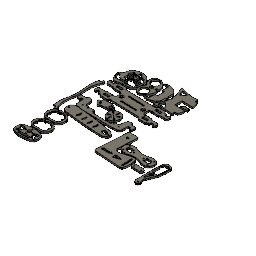
cat (Autodesk Fusion 360 design; units mm, degrees)
Autodesk Fusion 360 part; units mm, degrees
note: some values were not read from the file. Set by a fixed rule: which sketch regions a step uses.
(part 1 of 8)
sketch "Sketch1" plane through (0, 0, 0) normal (0, 1, 0) x (1, 0, 0)
  spline S0 degree 3 poles (30.1007, -167.9411) (18.5284, -167.6813) (11.3297, -174.7657) (11.4241, -183.0193) knots 0 0 0 0 1 1 1 1
  spline S1 degree 2 poles (11.4241, -183.0193) (11.5507, -194.1027) (22.4385, -196.859) knots 0 0 0 1 1 1
  line L0 (22.4385, -196.859) -> (39.1149, -197.0671)
  spline S2 degree 2 poles (39.1149, -197.0671) (49.0605, -194.4346) (48.8809, -182.6793) knots 0 0 0 1 1 1
  spline S3 degree 3 poles (48.8809, -182.6793) (48.7831, -176.2778) (41.5132, -168.2292) (30.1007, -167.9411) knots 0 0 0 0 1 1 1 1
  spline S4 degree 2 poles (16.3262, -186.15) (16.3682, -187.7873) (16.3594, -188.6061) knots 0 0 0 1 1 1
  spline S5 degree 3 poles (16.3594, -188.6061) (16.3555, -188.96) (16.5341, -189.4138) (17.0331, -189.4233) knots 0 0 0 0 1 1 1 1
  spline S6 degree 2 poles (17.0331, -189.4233) (17.5465, -189.433) (18.5735, -189.4411) knots 0 0 0 1 1 1
  spline S7 degree 2 poles (18.5735, -189.4411) (18.5349, -191.4596) (18.5681, -192.6548) knots 0 0 0 1 1 1
  spline S8 degree 3 poles (18.5681, -192.6548) (18.5726, -192.8153) (18.7396, -193.0355) (18.9408, -193.0336) knots 0 0 0 0 1 1 1 1
  spline S9 degree 3 poles (18.9408, -193.0336) (20.2717, -193.0206) (33.282, -192.9942) (40.4733, -192.9561) knots 0 0 0 0 1 1 1 1
  spline S10 degree 3 poles (40.4733, -192.9561) (40.6565, -192.9551) (40.8487, -192.7855) (40.8532, -192.6394) knots 0 0 0 0 1 1 1 1
  spline S11 degree 3 poles (40.8532, -192.6394) (40.8827, -191.6807) (40.867, -191.3134) (40.8652, -190.4928) knots 0 0 0 0 1 1 1 1
  spline S12 degree 3 poles (40.8652, -190.4928) (40.8648, -190.322) (41.0647, -190.1082) (41.2786, -190.1006) knots 0 0 0 0 1 1 1 1
  spline S13 degree 2 poles (41.2786, -190.1006) (41.9764, -190.0758) (43.3093, -190.0656) knots 0 0 0 1 1 1
  line L1 (43.3093, -190.0656) -> (43.2511, -186.7175)
  spline S14 degree 2 poles (43.2511, -186.7175) (41.3833, -185.9275) (41.4303, -183.8853) knots 0 0 0 1 1 1
  spline S15 degree 2 poles (41.4303, -183.8853) (41.4654, -182.3626) (43.665, -181.4955) knots 0 0 0 1 1 1
  line L2 (43.665, -181.4955) -> (43.6777, -178.3696)
  line L3 (43.6777, -178.3696) -> (41.9176, -178.351)
  spline S16 degree 3 poles (41.9176, -178.351) (41.6673, -178.3482) (41.388, -178.1253) (41.3891, -177.9256) knots 0 0 0 0 1 1 1 1
  line L4 (41.3891, -177.9256) -> (41.4058, -175.2138)
  spline S17 degree 3 poles (41.4058, -175.2138) (41.4074, -174.9545) (41.0839, -174.6323) (40.7588, -174.6317) knots 0 0 0 0 1 1 1 1
  line L5 (40.7588, -174.6317) -> (37.4248, -174.625)
  spline S18 degree 2 poles (37.4248, -174.625) (37.4304, -174.643) (37.4477, -173.8298) knots 0 0 0 1 1 1
  spline S19 degree 3 poles (37.4477, -173.8298) (37.4575, -173.3685) (37.471, -172.6397) (37.4893, -171.4884) knots 0 0 0 0 1 1 1 1
  spline S20 degree 3 poles (37.4893, -171.4884) (37.4915, -171.3464) (37.2058, -171.2102) (37.0279, -171.2118) knots 0 0 0 0 1 1 1 1
  spline S21 degree 3 poles (37.0279, -171.2118) (34.0609, -171.2378) (29.7217, -171.2387) (28.7942, -171.2468) knots 0 0 0 0 1 1 1 1
  spline S22 degree 3 poles (28.7942, -171.2468) (28.592, -171.2487) (28.1312, -171.3775) (28.1295, -171.5388) knots 0 0 0 0 1 1 1 1
  spline S23 degree 3 poles (28.1295, -171.5388) (28.1098, -173.3866) (28.1519, -172.4662) (28.1098, -173.3866) knots 0 0 0 0 1 1 1 1
  spline S24 degree 3 poles (28.1098, -173.3866) (28.0952, -173.7064) (27.5382, -174.0379) (27.2259, -174.0384) knots 0 0 0 0 1 1 1 1
  spline S25 degree 3 poles (27.2259, -174.0384) (25.0158, -174.0422) (22.0838, -174.0194) (20.0803, -174.0317) knots 0 0 0 0 1 1 1 1
  spline S26 degree 3 poles (20.0803, -174.0317) (19.6876, -174.0346) (19.3849, -174.3251) (19.3885, -174.6384) knots 0 0 0 0 1 1 1 1
  spline S27 degree 3 poles (19.3885, -174.6384) (19.3931, -175.0333) (19.3962, -176.3013) (19.4093, -176.8891) knots 0 0 0 0 1 1 1 1
  spline S28 degree 3 poles (19.4093, -176.8891) (19.4223, -177.4769) (19.0429, -177.3787) (18.7383, -177.3844) knots 0 0 0 0 1 1 1 1
  spline S29 degree 3 poles (18.7383, -177.3844) (18.0475, -177.3973) (17.5642, -177.4064) (17.2536, -177.4122) knots 0 0 0 0 1 1 1 1
  spline S30 degree 3 poles (17.2536, -177.4122) (16.943, -177.4179) (16.8656, -177.5739) (16.8603, -177.7204) knots 0 0 0 0 1 1 1 1
  spline S31 degree 2 poles (16.8603, -177.7204) (16.8284, -178.6066) (16.8714, -179.9909) knots 0 0 0 1 1 1
  spline S32 degree 3 poles (16.8714, -179.9909) (18.5933, -180.665) (18.7033, -181.7831) (18.7467, -183.0137) knots 0 0 0 0 1 1 1 1
  spline S33 degree 3 poles (18.7467, -183.0137) (18.7915, -184.2826) (18.3153, -185.8023) (16.3262, -186.15) knots 0 0 0 0 1 1 1 1
  spline S34 degree 3 poles (16.5132, -182.6529) (15.9028, -182.6481) (15.6342, -183.0282) (15.649, -183.3882) knots 0 0 0 0 1 1 1 1
  spline S35 degree 3 poles (15.649, -183.3882) (15.6637, -183.749) (15.9951, -184.0326) (16.5484, -184.0283) knots 0 0 0 0 1 1 1 1
  spline S36 degree 3 poles (16.5484, -184.0283) (17.0419, -184.0245) (17.3667, -183.6763) (17.3661, -183.3666) knots 0 0 0 0 1 1 1 1
  spline S37 degree 3 poles (17.3661, -183.3666) (17.3652, -182.9178) (16.9336, -182.6565) (16.5132, -182.6529) knots 0 0 0 0 1 1 1 1
  spline S38 degree 3 poles (43.0664, -183.5551) (42.456, -183.5503) (42.1875, -183.9304) (42.2022, -184.2904) knots 0 0 0 0 1 1 1 1
  spline S39 degree 3 poles (42.2022, -184.2904) (42.217, -184.6513) (42.5483, -184.9349) (43.1016, -184.9305) knots 0 0 0 0 1 1 1 1
  spline S40 degree 3 poles (43.1016, -184.9305) (43.5952, -184.9267) (43.9199, -184.5786) (43.9193, -184.2688) knots 0 0 0 0 1 1 1 1
  spline S41 degree 3 poles (43.9193, -184.2688) (43.9185, -183.8201) (43.4868, -183.5587) (43.0664, -183.5551) knots 0 0 0 0 1 1 1 1
  spline S42 degree 3 poles (23.7842, -171.0421) (22.7975, -171.0345) (22.3635, -171.6745) (22.3872, -172.281) knots 0 0 0 0 1 1 1 1
  spline S43 degree 3 poles (22.3872, -172.281) (22.4111, -172.889) (22.9467, -173.3668) (23.8411, -173.3594) knots 0 0 0 0 1 1 1 1
  spline S44 degree 3 poles (23.8411, -173.3594) (24.6388, -173.3528) (25.1637, -172.7664) (25.1628, -172.2446) knots 0 0 0 0 1 1 1 1
  spline S45 degree 3 poles (25.1628, -172.2446) (25.1615, -171.4885) (24.4637, -171.0481) (23.7842, -171.0421) knots 0 0 0 0 1 1 1 1
  spline S46 degree 3 poles (197.2264, -186.8151) (204.2093, -186.9093) (204.3289, -186.987) (213.7082, -187.3044) knots 0 0 0 0 1 1 1 1
  spline S47 degree 3 poles (213.7082, -187.3044) (214.9527, -187.2349) (217.7236, -188.5503) (217.578, -192.0838) knots 0 0 0 0 1 1 1 1
  spline S48 degree 3 poles (217.578, -192.0838) (217.428, -195.7284) (214.5453, -196.5174) (213.4322, -196.3773) knots 0 0 0 0 1 1 1 1
  spline S49 degree 3 poles (213.4322, -196.3773) (204.6722, -196.078) (204.6859, -195.9838) (197.5085, -195.7356) knots 0 0 0 0 1 1 1 1
  spline S50 degree 3 poles (197.5085, -195.7356) (196.2722, -195.7521) (193.3363, -194.4697) (193.4517, -191.1659) knots 0 0 0 0 1 1 1 1
  spline S51 degree 3 poles (193.4517, -191.1659) (193.5843, -187.3752) (195.8081, -186.9513) (197.2264, -186.8151) knots 0 0 0 0 1 1 1 1
  spline S52 degree 3 poles (197.9729, -187.867) (199.884, -187.9236) (201.1067, -189.5978) (201.0786, -191.1557) knots 0 0 0 0 1 1 1 1
  spline S53 degree 3 poles (201.0786, -191.1557) (201.0504, -192.8262) (199.5544, -194.4019) (197.7982, -194.3846) knots 0 0 0 0 1 1 1 1
  spline S54 degree 3 poles (197.7982, -194.3846) (196.0791, -194.3681) (194.5964, -192.8234) (194.5755, -191.0496) knots 0 0 0 0 1 1 1 1
  spline S55 degree 3 poles (194.5755, -191.0496) (194.5553, -189.4029) (195.9362, -187.8065) (197.9729, -187.867) knots 0 0 0 0 1 1 1 1
  spline S56 degree 3 poles (197.8992, -188.8932) (199.2233, -188.9345) (200.0706, -190.1307) (200.051, -191.2446) knots 0 0 0 0 1 1 1 1
  spline S57 degree 3 poles (200.051, -191.2446) (200.0267, -192.4391) (198.9949, -193.5657) (197.7781, -193.5533) knots 0 0 0 0 1 1 1 1
  spline S58 degree 3 poles (197.7781, -193.5533) (196.5871, -193.5409) (195.5596, -192.4371) (195.5452, -191.1688) knots 0 0 0 0 1 1 1 1
  spline S59 degree 3 poles (195.5452, -191.1688) (195.529, -189.9915) (196.4879, -188.85) (197.8992, -188.8932) knots 0 0 0 0 1 1 1 1
  spline S60 degree 3 poles (212.9873, -188.7216) (214.8985, -188.7782) (216.1212, -190.4524) (216.0931, -192.0102) knots 0 0 0 0 1 1 1 1
  spline S61 degree 3 poles (216.0931, -192.0102) (216.0648, -193.6808) (214.5689, -195.2565) (212.8127, -195.2392) knots 0 0 0 0 1 1 1 1
  spline S62 degree 3 poles (212.8127, -195.2392) (211.0936, -195.2227) (209.6108, -193.678) (209.59, -191.9042) knots 0 0 0 0 1 1 1 1
  spline S63 degree 3 poles (209.59, -191.9042) (209.5698, -190.2575) (210.9506, -188.6611) (212.9873, -188.7216) knots 0 0 0 0 1 1 1 1
  spline S64 degree 3 poles (212.9137, -189.7478) (214.2378, -189.7891) (215.0851, -190.9853) (215.0655, -192.0992) knots 0 0 0 0 1 1 1 1
  spline S65 degree 3 poles (215.0655, -192.0992) (215.0412, -193.2937) (214.0094, -194.4203) (212.7926, -194.4079) knots 0 0 0 0 1 1 1 1
  spline S66 degree 3 poles (212.7926, -194.4079) (211.6015, -194.3955) (210.5741, -193.2917) (210.5596, -192.0234) knots 0 0 0 0 1 1 1 1
  spline S67 degree 3 poles (210.5596, -192.0234) (210.5435, -190.8461) (211.5024, -189.7046) (212.9137, -189.7478) knots 0 0 0 0 1 1 1 1
  spline S68 degree 3 poles (197.9022, -190.3368) (198.3782, -190.3493) (198.6826, -190.771) (198.6756, -191.1619) knots 0 0 0 0 1 1 1 1
  spline S69 degree 3 poles (198.6756, -191.1619) (198.6674, -191.581) (198.296, -191.9763) (197.8586, -191.972) knots 0 0 0 0 1 1 1 1
  spline S70 degree 3 poles (197.8586, -191.972) (197.4305, -191.969) (197.0612, -191.5805) (197.056, -191.1353) knots 0 0 0 0 1 1 1 1
  spline S71 degree 3 poles (197.056, -191.1353) (197.0479, -190.7223) (197.3951, -190.3217) (197.9022, -190.3368) knots 0 0 0 0 1 1 1 1
  spline S72 degree 3 poles (212.9168, -191.2402) (213.3928, -191.2526) (213.6972, -191.6744) (213.6902, -192.0653) knots 0 0 0 0 1 1 1 1
  spline S73 degree 3 poles (213.6902, -192.0653) (213.682, -192.4843) (213.3106, -192.8796) (212.8732, -192.8753) knots 0 0 0 0 1 1 1 1
  spline S74 degree 3 poles (212.8732, -192.8753) (212.4451, -192.8723) (212.0758, -192.4838) (212.0706, -192.0386) knots 0 0 0 0 1 1 1 1
  spline S75 degree 3 poles (212.0706, -192.0386) (212.0625, -191.6256) (212.4097, -191.2251) (212.9168, -191.2402) knots 0 0 0 0 1 1 1 1
  line L6 (146.865, -211.1125) -> (145.6182, -211.0016)
  spline S76 degree 3 poles (145.6182, -211.0016) (143.5328, -215.233) (142.4397, -219.9965) (142.4613, -224.7587) knots 0 0 0 0 1 1 1 1
  spline S77 degree 3 poles (142.4613, -224.7587) (142.4822, -229.3508) (143.5381, -233.9343) (145.519, -238.0307) knots 0 0 0 0 1 1 1 1
  line L7 (145.519, -238.0307) -> (146.5081, -237.9343)
  line L8 (146.5081, -237.9343) -> (147.1109, -234.9727)
  line L9 (147.1109, -234.9727) -> (150.1451, -235.1898)
  line L10 (150.1451, -235.1898) -> (150.4167, -238.3519)
  spline S78 degree 3 poles (150.4167, -238.3519) (151.2044, -238.3226) (151.9926, -238.3081) (152.7808, -238.3082) knots 0 0 0 0 1 1 1 1
  spline S79 degree 3 poles (152.7808, -238.3082) (155.0336, -238.3085) (157.3099, -238.4326) (159.4772, -239.077) knots 0 0 0 0 1 1 1 1
  spline S80 degree 3 poles (159.4772, -239.077) (162.8464, -240.0787) (165.767, -242.276) (168.9964, -243.6958) knots 0 0 0 0 1 1 1 1
  spline S81 degree 3 poles (168.9964, -243.6958) (172.6327, -245.2945) (176.6166, -245.8823) (180.56, -245.9048) knots 0 0 0 0 1 1 1 1
  spline S82 degree 3 poles (180.56, -245.9048) (184.3344, -245.9265) (188.147, -245.4327) (191.6764, -244.0305) knots 0 0 0 0 1 1 1 1
  spline S83 degree 3 poles (191.6764, -244.0305) (195.8908, -242.3562) (199.6632, -239.411) (204.0862, -238.5023) knots 0 0 0 0 1 1 1 1
  spline S84 degree 3 poles (204.0862, -238.5023) (205.3946, -238.2335) (206.7377, -238.1508) (208.0672, -238.2572) knots 0 0 0 0 1 1 1 1
  line L11 (208.0672, -238.2572) -> (210.3957, -238.4357)
  line L12 (210.3957, -238.4357) -> (210.8097, -235.2303)
  line L13 (210.8097, -235.2303) -> (213.5445, -235.2773)
  line L14 (213.5445, -235.2773) -> (214.0524, -237.8947)
  line L15 (214.0524, -237.8947) -> (215.7016, -237.8617)
  spline S85 degree 3 poles (215.7016, -237.8617) (216.1906, -236.8171) (216.6159, -235.7396) (216.9738, -234.6382) knots 0 0 0 0 1 1 1 1
  spline S86 degree 3 poles (216.9738, -234.6382) (218.027, -231.3975) (218.4906, -227.9675) (218.5697, -224.5451) knots 0 0 0 0 1 1 1 1
  spline S87 degree 3 poles (218.5697, -224.5451) (218.6361, -221.6728) (218.4324, -218.7783) (217.7433, -215.9974) knots 0 0 0 0 1 1 1 1
  spline S88 degree 3 poles (217.7433, -215.9974) (217.3137, -214.2641) (216.6969, -212.5818) (215.9083, -210.993) knots 0 0 0 0 1 1 1 1
  line L16 (215.9083, -210.993) -> (214.1259, -211.0241)
  line L17 (214.1259, -211.0241) -> (213.9265, -214.1277)
  line L18 (213.9265, -214.1277) -> (210.6322, -213.958)
  spline S89 degree 3 poles (210.6322, -213.958) (210.5729, -213.3726) (210.5658, -212.7815) (210.611, -212.1948) knots 0 0 0 0 1 1 1 1
  spline S90 degree 3 poles (210.611, -212.1948) (210.6283, -211.9695) (210.6533, -211.743) (210.6307, -211.5182) knots 0 0 0 0 1 1 1 1
  spline S91 degree 3 poles (210.6307, -211.5182) (210.608, -211.2935) (210.5323, -211.0664) (210.3768, -210.9098) knots 0 0 0 0 1 1 1 1
  spline S92 degree 3 poles (210.3768, -210.9098) (210.2363, -210.7684) (210.0354, -210.6956) (209.8416, -210.7158) knots 0 0 0 0 1 1 1 1
  spline S93 degree 3 poles (209.8416, -210.7158) (209.6478, -210.736) (209.4646, -210.8489) (209.3535, -211.0165) knots 0 0 0 0 1 1 1 1
  spline S94 degree 3 poles (209.3535, -211.0165) (206.6023, -213.213) (202.9, -214.0441) (199.5315, -213.2216) knots 0 0 0 0 1 1 1 1
  spline S95 degree 3 poles (199.5315, -213.2216) (197.267, -212.6687) (195.2184, -211.4328) (193.0787, -210.4795) knots 0 0 0 0 1 1 1 1
  spline S96 degree 3 poles (193.0787, -210.4795) (189.1673, -208.737) (184.8924, -207.9308) (180.6427, -208.0084) knots 0 0 0 0 1 1 1 1
  spline S97 degree 3 poles (180.6427, -208.0084) (176.3537, -208.0868) (172.1019, -209.0544) (168.0772, -210.6096) knots 0 0 0 0 1 1 1 1
  spline S98 degree 3 poles (168.0772, -210.6096) (164.8763, -211.8464) (161.7028, -213.4776) (158.2919, -213.5448) knots 0 0 0 0 1 1 1 1
  spline S99 degree 3 poles (158.2919, -213.5448) (156.5255, -213.5795) (154.6945, -213.1518) (153.3097, -212.0024) knots 0 0 0 0 1 1 1 1
  spline S100 degree 3 poles (153.3097, -212.0024) (153.0083, -211.7523) (152.7298, -211.4699) (152.4066, -211.2518) knots 0 0 0 0 1 1 1 1
  spline S101 degree 3 poles (152.4066, -211.2518) (152.0833, -211.0337) (151.7007, -210.8809) (151.3189, -210.9292) knots 0 0 0 0 1 1 1 1
  spline S102 degree 3 poles (151.3189, -210.9292) (151.021, -210.9669) (150.7394, -211.1305) (150.5511, -211.3753) knots 0 0 0 0 1 1 1 1
  spline S103 degree 3 poles (150.5511, -211.3753) (150.3629, -211.6201) (150.2701, -211.9432) (150.2982, -212.2562) knots 0 0 0 0 1 1 1 1
  line L19 (150.2982, -212.2562) -> (150.1937, -214.0445)
  line L20 (150.1937, -214.0445) -> (146.9587, -214.0134)
  line L21 (146.9587, -214.0134) -> (146.865, -211.1125)
  line L22 (175.7677, -213.3062) -> (185.4169, -213.3732)
  spline S104 degree 3 poles (185.4169, -213.3732) (185.5698, -213.3654) (185.7249, -213.4272) (185.8333, -213.5405) knots 0 0 0 0 1 1 1 1
  spline S105 degree 3 poles (185.8333, -213.5405) (185.9415, -213.6536) (186.0014, -213.8157) (185.9941, -213.9756) knots 0 0 0 0 1 1 1 1
  line L23 (185.9941, -213.9756) -> (185.9941, -235.4239)
  spline S106 degree 3 poles (185.9941, -235.4239) (185.9786, -235.596) (185.9102, -235.7625) (185.8013, -235.8925) knots 0 0 0 0 1 1 1 1
  spline S107 degree 3 poles (185.8013, -235.8925) (185.6858, -236.0305) (185.5252, -236.1263) (185.353, -236.1602) knots 0 0 0 0 1 1 1 1
  line L24 (185.353, -236.1602) -> (175.8327, -235.9594)
  spline S108 degree 3 poles (175.8327, -235.9594) (175.6725, -235.8987) (175.5277, -235.7938) (175.4169, -235.6581) knots 0 0 0 0 1 1 1 1
  spline S109 degree 3 poles (175.4169, -235.6581) (175.3008, -235.516) (175.2225, -235.3405) (175.1927, -235.1561) knots 0 0 0 0 1 1 1 1
  line L25 (175.1927, -235.1561) -> (175.1608, -213.9224)
  spline S110 degree 3 poles (175.1608, -213.9224) (175.1845, -213.7836) (175.2461, -213.652) (175.3365, -213.5474) knots 0 0 0 0 1 1 1 1
  spline S111 degree 3 poles (175.3365, -213.5474) (175.448, -213.4183) (175.6033, -213.3315) (175.7677, -213.3062) knots 0 0 0 0 1 1 1 1
  line L26 (163.9244, -228.8555) -> (163.9212, -233.8159)
  spline S112 degree 3 poles (163.9212, -233.8159) (163.875, -234.1512) (163.9842, -234.5062) (164.2085, -234.7502) knots 0 0 0 0 1 1 1 1
  spline S113 degree 3 poles (164.2085, -234.7502) (164.3318, -234.8843) (164.4876, -234.9853) (164.6572, -235.041) knots 0 0 0 0 1 1 1 1
  spline S114 degree 3 poles (164.6572, -235.041) (164.8268, -235.0967) (165.0097, -235.107) (165.184, -235.0706) knots 0 0 0 0 1 1 1 1
  line L27 (165.184, -235.0706) -> (171.8437, -235.1161)
  spline S115 degree 3 poles (171.8437, -235.1161) (172.1006, -235.0921) (172.345, -234.9471) (172.4969, -234.7287) knots 0 0 0 0 1 1 1 1
  spline S116 degree 3 poles (172.4969, -234.7287) (172.6109, -234.5648) (172.6729, -234.3619) (172.6711, -234.1591) knots 0 0 0 0 1 1 1 1
  line L28 (172.6711, -234.1591) -> (172.6914, -228.797)
  spline S117 degree 3 poles (172.6914, -228.797) (172.692, -228.6495) (172.6925, -228.5015) (172.6735, -228.3554) knots 0 0 0 0 1 1 1 1
  spline S118 degree 3 poles (172.6735, -228.3554) (172.6542, -228.2093) (172.6138, -228.064) (172.5361, -227.941) knots 0 0 0 0 1 1 1 1
  spline S119 degree 3 poles (172.5361, -227.941) (172.465, -227.8286) (172.3636, -227.7375) (172.2466, -227.6812) knots 0 0 0 0 1 1 1 1
  spline S120 degree 3 poles (172.2466, -227.6812) (172.1296, -227.6249) (171.9975, -227.6037) (171.8698, -227.6206) knots 0 0 0 0 1 1 1 1
  line L29 (171.8698, -227.6206) -> (164.5904, -227.6875)
  spline S121 degree 3 poles (164.5904, -227.6875) (164.3694, -227.7576) (164.1743, -227.9139) (164.0518, -228.1191) knots 0 0 0 0 1 1 1 1
  spline S122 degree 3 poles (164.0518, -228.1191) (163.9225, -228.3357) (163.8758, -228.605) (163.9244, -228.8555) knots 0 0 0 0 1 1 1 1
  line L30 (187.9184, -228.9748) -> (188.0011, -233.9299)
  spline S123 degree 3 poles (188.0011, -233.9299) (188.0279, -234.2742) (188.1865, -234.6053) (188.4341, -234.8334) knots 0 0 0 0 1 1 1 1
  spline S124 degree 3 poles (188.4341, -234.8334) (188.6573, -235.039) (188.9502, -235.1598) (189.2473, -235.1688) knots 0 0 0 0 1 1 1 1
  line L31 (189.2473, -235.1688) -> (196.0874, -235.1491)
  spline S125 degree 3 poles (196.0874, -235.1491) (196.4065, -235.1391) (196.7165, -234.9587) (196.8928, -234.6798) knots 0 0 0 0 1 1 1 1
  spline S126 degree 3 poles (196.8928, -234.6798) (196.9656, -234.5647) (197.0157, -234.4345) (197.0428, -234.2994) knots 0 0 0 0 1 1 1 1
  spline S127 degree 3 poles (197.0428, -234.2994) (197.0699, -234.1643) (197.073, -234.0254) (197.0735, -233.8873) knots 0 0 0 0 1 1 1 1
  line L32 (197.0735, -233.8873) -> (197.0923, -228.9078)
  spline S128 degree 3 poles (197.0923, -228.9078) (197.0727, -228.5996) (196.9287, -228.3023) (196.7028, -228.1038) knots 0 0 0 0 1 1 1 1
  spline S129 degree 3 poles (196.7028, -228.1038) (196.5063, -227.9312) (196.2504, -227.8342) (195.9939, -227.8354) knots 0 0 0 0 1 1 1 1
  line L33 (195.9939, -227.8354) -> (188.9046, -227.8076)
  spline S130 degree 3 poles (188.9046, -227.8076) (188.7383, -227.801) (188.5704, -227.8396) (188.4227, -227.9201) knots 0 0 0 0 1 1 1 1
  spline S131 degree 3 poles (188.4227, -227.9201) (188.275, -228.0006) (188.1479, -228.122) (188.0579, -228.2688) knots 0 0 0 0 1 1 1 1
  spline S132 degree 3 poles (188.0579, -228.2688) (187.9312, -228.4756) (187.8805, -228.7322) (187.9184, -228.9748) knots 0 0 0 0 1 1 1 1
  line L34 (170.0186, -222.2752) -> (162.7994, -223.1454)
  spline S133 degree 3 poles (162.7994, -223.1454) (162.5278, -223.1766) (162.2457, -223.0903) (162.0327, -222.911) knots 0 0 0 0 1 1 1 1
  spline S134 degree 3 poles (162.0327, -222.911) (161.8968, -222.7967) (161.789, -222.6459) (161.7224, -222.4772) knots 0 0 0 0 1 1 1 1
  spline S135 degree 3 poles (161.7224, -222.4772) (161.6557, -222.3084) (161.6304, -222.122) (161.6494, -221.9404) knots 0 0 0 0 1 1 1 1
  line L35 (161.6494, -221.9404) -> (161.4651, -219.7207)
  spline S136 degree 3 poles (161.4651, -219.7207) (161.4358, -219.4894) (161.4927, -219.2472) (161.6212, -219.0566) knots 0 0 0 0 1 1 1 1
  spline S137 degree 3 poles (161.6212, -219.0566) (161.7857, -218.8127) (162.0671, -218.6601) (162.3522, -218.6604) knots 0 0 0 0 1 1 1 1
  line L36 (162.3522, -218.6604) -> (169.316, -217.6563)
  spline S138 degree 3 poles (169.316, -217.6563) (169.6522, -217.6146) (170.0024, -217.7125) (170.2742, -217.9241) knots 0 0 0 0 1 1 1 1
  spline S139 degree 3 poles (170.2742, -217.9241) (170.5631, -218.1489) (170.7593, -218.5001) (170.8051, -218.874) knots 0 0 0 0 1 1 1 1
  line L37 (170.8051, -218.874) -> (170.8732, -220.9866)
  spline S140 degree 3 poles (170.8732, -220.9866) (170.8785, -221.2891) (170.7825, -221.5925) (170.6057, -221.8317) knots 0 0 0 0 1 1 1 1
  spline S141 degree 3 poles (170.6057, -221.8317) (170.4559, -222.0343) (170.2494, -222.1903) (170.0186, -222.2752) knots 0 0 0 0 1 1 1 1
  line L38 (198.197, -223.3422) -> (191.3245, -221.9128)
  spline S142 degree 3 poles (191.3245, -221.9128) (191.0607, -221.8499) (190.821, -221.6821) (190.6647, -221.4508) knots 0 0 0 0 1 1 1 1
  spline S143 degree 3 poles (190.6647, -221.4508) (190.4638, -221.1537) (190.4074, -220.7548) (190.5174, -220.4095) knots 0 0 0 0 1 1 1 1
  line L39 (190.5174, -220.4095) -> (190.8221, -218.2444)
  spline S144 degree 3 poles (190.8221, -218.2444) (190.8379, -218.0208) (190.9439, -217.8057) (191.1088, -217.6628) knots 0 0 0 0 1 1 1 1
  spline S145 degree 3 poles (191.1088, -217.6628) (191.2127, -217.5728) (191.3388, -217.511) (191.4714, -217.4853) knots 0 0 0 0 1 1 1 1
  spline S146 degree 3 poles (191.4714, -217.4853) (191.604, -217.4595) (191.7429, -217.4698) (191.8707, -217.515) knots 0 0 0 0 1 1 1 1
  line L40 (191.8707, -217.515) -> (198.5352, -218.7375)
  spline S147 degree 3 poles (198.5352, -218.7375) (198.8622, -218.8129) (199.1617, -219.0127) (199.3654, -219.2912) knots 0 0 0 0 1 1 1 1
  spline S148 degree 3 poles (199.3654, -219.2912) (199.5853, -219.5919) (199.6906, -219.982) (199.6536, -220.3589) knots 0 0 0 0 1 1 1 1
  line L41 (199.6536, -220.3589) -> (199.2644, -222.3859)
  spline S149 degree 3 poles (199.2644, -222.3859) (199.2116, -222.6695) (199.0558, -222.9307) (198.8356, -223.1046) knots 0 0 0 0 1 1 1 1
  spline S150 degree 3 poles (198.8356, -223.1046) (198.6524, -223.2494) (198.4262, -223.3335) (198.197, -223.3422) knots 0 0 0 0 1 1 1 1
  spline S151 degree 3 poles (177.8923, -243.2372) (178.0147, -243.3291) (178.1552, -243.3939) (178.3018, -243.4299) knots 0 0 0 0 1 1 1 1
  spline S152 degree 3 poles (178.3018, -243.4299) (178.4484, -243.4659) (178.6001, -243.4715) (178.7507, -243.474) knots 0 0 0 0 1 1 1 1
  line L42 (178.7507, -243.474) -> (181.8525, -243.5228)
  spline S153 degree 3 poles (181.8525, -243.5228) (182.2174, -243.5104) (182.5745, -243.3344) (182.8164, -243.048) knots 0 0 0 0 1 1 1 1
  spline S154 degree 3 poles (182.8164, -243.048) (183.0715, -242.746) (183.1936, -242.3239) (183.1352, -241.9253) knots 0 0 0 0 1 1 1 1
  spline S155 degree 3 poles (183.1352, -241.9253) (183.0769, -241.5267) (182.8371, -241.1603) (182.5002, -240.9653) knots 0 0 0 0 1 1 1 1
  spline S156 degree 3 poles (182.5002, -240.9653) (182.255, -240.8234) (181.963, -240.7724) (181.687, -240.8233) knots 0 0 0 0 1 1 1 1
  line L43 (181.687, -240.8233) -> (178.6725, -240.775)
  spline S157 degree 3 poles (178.6725, -240.775) (178.5266, -240.7728) (178.3792, -240.7755) (178.2379, -240.8133) knots 0 0 0 0 1 1 1 1
  spline S158 degree 3 poles (178.2379, -240.8133) (178.0966, -240.8512) (177.9639, -240.9211) (177.8472, -241.0127) knots 0 0 0 0 1 1 1 1
  spline S159 degree 3 poles (177.8472, -241.0127) (177.5162, -241.2721) (177.3152, -241.7042) (177.324, -242.1371) knots 0 0 0 0 1 1 1 1
  spline S160 degree 3 poles (177.324, -242.1371) (177.3325, -242.5701) (177.5511, -242.9928) (177.8923, -243.2372) knots 0 0 0 0 1 1 1 1
  spline S161 degree 3 poles (180.3317, -237.7466) (180.0656, -237.7578) (179.7785, -238.083) (179.7896, -238.3619) knots 0 0 0 0 1 1 1 1
  spline S162 degree 3 poles (179.7896, -238.3619) (179.8002, -238.6185) (180.0866, -238.883) (180.3317, -238.8825) knots 0 0 0 0 1 1 1 1
  spline S163 degree 3 poles (180.3317, -238.8825) (180.5981, -238.8821) (180.919, -238.5937) (180.919, -238.3146) knots 0 0 0 0 1 1 1 1
  spline S164 degree 3 poles (180.919, -238.3146) (180.919, -238.0354) (180.5979, -237.7354) (180.3317, -237.7466) knots 0 0 0 0 1 1 1 1
  spline S165 degree 3 poles (180.5804, -210.3406) (180.3142, -210.3518) (180.0272, -210.677) (180.0383, -210.9559) knots 0 0 0 0 1 1 1 1
  spline S166 degree 3 poles (180.0383, -210.9559) (180.0489, -211.2125) (180.3353, -211.477) (180.5804, -211.4766) knots 0 0 0 0 1 1 1 1
  spline S167 degree 3 poles (180.5804, -211.4766) (180.8468, -211.4761) (181.1677, -211.1877) (181.1677, -210.9086) knots 0 0 0 0 1 1 1 1
  spline S168 degree 3 poles (181.1677, -210.9086) (181.1677, -210.6295) (180.8466, -210.3294) (180.5804, -210.3406) knots 0 0 0 0 1 1 1 1
  spline S169 degree 3 poles (87.8377, -110.5872) (84.4918, -110.7696) (81.236, -112.3681) (79.0016, -114.9427) knots 0 0 0 0 1 1 1 1
  spline S170 degree 3 poles (79.0016, -114.9427) (76.7673, -117.5174) (75.5862, -121.0383) (75.8169, -124.4851) knots 0 0 0 0 1 1 1 1
  spline S171 degree 3 poles (75.8169, -124.4851) (76.0391, -127.8061) (77.5645, -131.0121) (79.9651, -133.2378) knots 0 0 0 0 1 1 1 1
  spline S172 degree 3 poles (79.9651, -133.2378) (82.3657, -135.4635) (85.6124, -136.6872) (88.8395, -136.5989) knots 0 0 0 0 1 1 1 1
  spline S173 degree 3 poles (88.8395, -136.5989) (92.1214, -136.509) (95.3527, -135.0611) (97.6441, -132.6368) knots 0 0 0 0 1 1 1 1
  spline S174 degree 3 poles (97.6441, -132.6368) (99.9355, -130.2124) (101.2572, -126.8374) (101.2246, -123.4522) knots 0 0 0 0 1 1 1 1
  spline S175 degree 3 poles (101.2246, -123.4522) (101.1908, -119.9384) (99.6936, -116.468) (97.1968, -114.0765) knots 0 0 0 0 1 1 1 1
  spline S176 degree 3 poles (97.1968, -114.0765) (94.7, -111.6849) (91.2408, -110.4016) (87.8377, -110.5872) knots 0 0 0 0 1 1 1 1
  line L44 (84.5138, -120.8698) -> (80.3813, -118.6573)
  spline S177 degree 3 poles (80.3813, -118.6573) (80.0801, -118.4223) (79.8836, -118.05) (79.8558, -117.6616) knots 0 0 0 0 1 1 1 1
  spline S178 degree 3 poles (79.8558, -117.6616) (79.828, -117.2732) (79.9692, -116.8752) (80.2336, -116.5971) knots 0 0 0 0 1 1 1 1
  spline S179 degree 3 poles (80.2336, -116.5971) (80.4902, -116.3272) (80.8585, -116.1741) (81.225, -116.185) knots 0 0 0 0 1 1 1 1
  spline S180 degree 3 poles (81.225, -116.185) (81.5914, -116.196) (81.9505, -116.3707) (82.1916, -116.6555) knots 0 0 0 0 1 1 1 1
  line L45 (82.1916, -116.6555) -> (84.9102, -120.3218)
  spline S181 degree 3 poles (84.9102, -120.3218) (84.9596, -120.3668) (84.9955, -120.4273) (85.012, -120.4931) knots 0 0 0 0 1 1 1 1
  spline S182 degree 3 poles (85.012, -120.4931) (85.0284, -120.5589) (85.0254, -120.6297) (85.0032, -120.6937) knots 0 0 0 0 1 1 1 1
  spline S183 degree 3 poles (85.0032, -120.6937) (84.97, -120.79) (84.8929, -120.869) (84.7994, -120.9026) knots 0 0 0 0 1 1 1 1
  spline S184 degree 3 poles (84.7994, -120.9026) (84.7058, -120.9362) (84.5978, -120.9239) (84.5138, -120.8698) knots 0 0 0 0 1 1 1 1
  spline S185 degree 3 poles (95.6513, -128.1996) (95.9444, -128.379) (96.165, -128.6802) (96.2523, -129.0199) knots 0 0 0 0 1 1 1 1
  spline S186 degree 3 poles (96.2523, -129.0199) (96.3396, -129.3597) (96.2926, -129.734) (96.1241, -130.0396) knots 0 0 0 0 1 1 1 1
  spline S187 degree 3 poles (96.1241, -130.0396) (95.9293, -130.393) (95.5731, -130.647) (95.1836, -130.7103) knots 0 0 0 0 1 1 1 1
  spline S188 degree 3 poles (95.1836, -130.7103) (94.7941, -130.7737) (94.3795, -130.6448) (94.0887, -130.3703) knots 0 0 0 0 1 1 1 1
  line L46 (94.0887, -130.3703) -> (91.2541, -126.7052)
  spline S189 degree 3 poles (91.2541, -126.7052) (91.2029, -126.6418) (91.1738, -126.5599) (91.173, -126.4774) knots 0 0 0 0 1 1 1 1
  spline S190 degree 3 poles (91.173, -126.4774) (91.1723, -126.395) (91.2, -126.3125) (91.25, -126.2481) knots 0 0 0 0 1 1 1 1
  spline S191 degree 3 poles (91.25, -126.2481) (91.3094, -126.1718) (91.3999, -126.1222) (91.4945, -126.1141) knots 0 0 0 0 1 1 1 1
  spline S192 degree 3 poles (91.4945, -126.1141) (91.589, -126.1064) (91.6863, -126.1397) (91.757, -126.205) knots 0 0 0 0 1 1 1 1
  line L47 (91.757, -126.205) -> (95.6513, -128.1996)
  spline S193 degree 3 poles (95.9911, -119.2601) (96.2564, -119.0604) (96.6058, -118.9842) (96.9269, -119.0559) knots 0 0 0 0 1 1 1 1
  spline S194 degree 3 poles (96.9269, -119.0559) (97.2479, -119.1276) (97.5354, -119.3461) (97.6969, -119.6411) knots 0 0 0 0 1 1 1 1
  spline S195 degree 3 poles (97.6969, -119.6411) (97.8559, -119.9317) (97.8903, -120.2917) (97.7895, -120.6087) knots 0 0 0 0 1 1 1 1
  spline S196 degree 3 poles (97.7895, -120.6087) (97.6886, -120.9257) (97.454, -121.1947) (97.159, -121.3316) knots 0 0 0 0 1 1 1 1
  line L48 (97.159, -121.3316) -> (92.6906, -122.4058)
  spline S197 degree 3 poles (92.6906, -122.4058) (92.6145, -122.4329) (92.5295, -122.4329) (92.4534, -122.4057) knots 0 0 0 0 1 1 1 1
  spline S198 degree 3 poles (92.4534, -122.4057) (92.3772, -122.3785) (92.3104, -122.3244) (92.2669, -122.2545) knots 0 0 0 0 1 1 1 1
  spline S199 degree 3 poles (92.2669, -122.2545) (92.2231, -122.1844) (92.2031, -122.0989) (92.2109, -122.016) knots 0 0 0 0 1 1 1 1
  spline S200 degree 3 poles (92.2109, -122.016) (92.2187, -121.933) (92.2543, -121.8531) (92.3103, -121.793) knots 0 0 0 0 1 1 1 1
  line L49 (92.3103, -121.793) -> (95.9911, -119.2601)
  spline S201 degree 3 poles (80.0987, -128.1123) (79.8187, -128.2317) (79.4945, -128.2368) (79.211, -128.1264) knots 0 0 0 0 1 1 1 1
  spline S202 degree 3 poles (79.211, -128.1264) (78.9275, -128.0159) (78.6876, -127.791) (78.554, -127.5105) knots 0 0 0 0 1 1 1 1
  spline S203 degree 3 poles (78.554, -127.5105) (78.4007, -127.1885) (78.3916, -126.7971) (78.5297, -126.4678) knots 0 0 0 0 1 1 1 1
  spline S204 degree 3 poles (78.5297, -126.4678) (78.6678, -126.1386) (78.9507, -125.8774) (79.2833, -125.7721) knots 0 0 0 0 1 1 1 1
  line L50 (79.2833, -125.7721) -> (83.8434, -124.8303)
  spline S205 degree 3 poles (83.8434, -124.8303) (83.9215, -124.7935) (84.013, -124.7877) (84.0948, -124.8145) knots 0 0 0 0 1 1 1 1
  spline S206 degree 3 poles (84.0948, -124.8145) (84.1766, -124.8413) (84.2481, -124.9004) (84.2912, -124.977) knots 0 0 0 0 1 1 1 1
  spline S207 degree 3 poles (84.2912, -124.977) (84.3347, -125.0543) (84.3489, -125.1487) (84.3302, -125.2359) knots 0 0 0 0 1 1 1 1
  spline S208 degree 3 poles (84.3302, -125.2359) (84.3114, -125.3233) (84.2599, -125.4025) (84.1888, -125.4536) knots 0 0 0 0 1 1 1 1
  line L51 (84.1888, -125.4536) -> (80.0987, -128.1123)
  line L52 (88.6963, -119.2519) -> (88.675, -114.4028)
  spline S209 degree 3 poles (88.675, -114.4028) (88.6406, -114.0553) (88.7574, -113.6949) (88.9875, -113.4385) knots 0 0 0 0 1 1 1 1
  spline S210 degree 3 poles (88.9875, -113.4385) (89.2176, -113.1822) (89.5571, -113.0343) (89.8957, -113.0428) knots 0 0 0 0 1 1 1 1
  spline S211 degree 3 poles (89.8957, -113.0428) (90.2902, -113.0527) (90.6737, -113.2784) (90.8826, -113.6236) knots 0 0 0 0 1 1 1 1
  spline S212 degree 3 poles (90.8826, -113.6236) (91.0916, -113.9689) (91.1196, -114.4233) (90.9549, -114.7931) knots 0 0 0 0 1 1 1 1
  line L53 (90.9549, -114.7931) -> (89.5024, -119.3859)
  spline S213 degree 3 poles (89.5024, -119.3859) (89.4846, -119.4831) (89.4322, -119.5733) (89.3575, -119.6355) knots 0 0 0 0 1 1 1 1
  spline S214 degree 3 poles (89.3575, -119.6355) (89.2828, -119.6976) (89.1863, -119.7313) (89.0903, -119.7287) knots 0 0 0 0 1 1 1 1
  spline S215 degree 3 poles (89.0903, -119.7287) (88.9762, -119.7254) (88.8643, -119.6705) (88.7902, -119.5809) knots 0 0 0 0 1 1 1 1
  spline S216 degree 3 poles (88.7902, -119.5809) (88.7162, -119.4913) (88.6811, -119.3687) (88.6963, -119.2519) knots 0 0 0 0 1 1 1 1
  spline S217 degree 3 poles (87.8977, -127.9601) (87.9089, -129.4698) (87.9162, -130.9795) (87.9196, -132.4893) knots 0 0 0 0 1 1 1 1
  spline S218 degree 3 poles (87.9196, -132.4893) (87.9274, -132.8282) (87.7934, -133.1682) (87.5586, -133.4055) knots 0 0 0 0 1 1 1 1
  spline S219 degree 3 poles (87.5586, -133.4055) (87.3238, -133.6429) (86.9916, -133.7742) (86.6631, -133.7595) knots 0 0 0 0 1 1 1 1
  spline S220 degree 3 poles (86.6631, -133.7595) (86.292, -133.7429) (85.9332, -133.538) (85.7227, -133.2224) knots 0 0 0 0 1 1 1 1
  spline S221 degree 3 poles (85.7227, -133.2224) (85.5123, -132.9068) (85.4551, -132.488) (85.5728, -132.1247) knots 0 0 0 0 1 1 1 1
  line L54 (85.5728, -132.1247) -> (87.0679, -127.8349)
  spline S222 degree 3 poles (87.0679, -127.8349) (87.0929, -127.7408) (87.1495, -127.6561) (87.2258, -127.5985) knots 0 0 0 0 1 1 1 1
  spline S223 degree 3 poles (87.2258, -127.5985) (87.3021, -127.5409) (87.3975, -127.5109) (87.492, -127.5147) knots 0 0 0 0 1 1 1 1
  spline S224 degree 3 poles (87.492, -127.5147) (87.6014, -127.5191) (87.7083, -127.5694) (87.7832, -127.6517) knots 0 0 0 0 1 1 1 1
  spline S225 degree 3 poles (87.7832, -127.6517) (87.8581, -127.734) (87.9001, -127.8471) (87.8977, -127.9601) knots 0 0 0 0 1 1 1 1
  spline S226 degree 3 poles (88.2976, -123.1479) (88.1746, -123.1402) (88.0492, -123.1865) (87.9591, -123.2731) knots 0 0 0 0 1 1 1 1
  spline S227 degree 3 poles (87.9591, -123.2731) (87.8691, -123.3598) (87.8155, -123.4856) (87.8147, -123.6127) knots 0 0 0 0 1 1 1 1
  spline S228 degree 3 poles (87.8147, -123.6127) (87.8139, -123.724) (87.8532, -123.8352) (87.9234, -123.9198) knots 0 0 0 0 1 1 1 1
  spline S229 degree 3 poles (87.9234, -123.9198) (87.9936, -124.0044) (88.0942, -124.0616) (88.201, -124.0775) knots 0 0 0 0 1 1 1 1
  spline S230 degree 3 poles (88.201, -124.0775) (88.3292, -124.0966) (88.4646, -124.055) (88.5619, -123.967) knots 0 0 0 0 1 1 1 1
  spline S231 degree 3 poles (88.5619, -123.967) (88.6593, -123.879) (88.717, -123.7462) (88.7162, -123.6127) knots 0 0 0 0 1 1 1 1
  spline S232 degree 3 poles (88.7162, -123.6127) (88.7155, -123.4966) (88.6713, -123.3814) (88.5947, -123.2963) knots 0 0 0 0 1 1 1 1
  spline S233 degree 3 poles (88.5947, -123.2963) (88.518, -123.2112) (88.4099, -123.1572) (88.2976, -123.1479) knots 0 0 0 0 1 1 1 1
  line L55 (145.2588, -33.5908) -> (147.4545, -33.5908)
  line L56 (147.4545, -33.5908) -> (147.4545, -34.5936)
  spline S234 degree 3 poles (147.4545, -34.5936) (147.4426, -34.7069) (147.4761, -34.8243) (147.5459, -34.9144) knots 0 0 0 0 1 1 1 1
  spline S235 degree 3 poles (147.5459, -34.9144) (147.6304, -35.0236) (147.7677, -35.0901) (147.9058, -35.0889) knots 0 0 0 0 1 1 1 1
  line L57 (147.9058, -35.0889) -> (150.9762, -35.0807)
  spline S236 degree 3 poles (150.9762, -35.0807) (151.1407, -35.0795) (151.3039, -35.0163) (151.4262, -34.9063) knots 0 0 0 0 1 1 1 1
  spline S237 degree 3 poles (151.4262, -34.9063) (151.56, -34.786) (151.6429, -34.6103) (151.6509, -34.4307) knots 0 0 0 0 1 1 1 1
  line L58 (151.6509, -34.4307) -> (151.6322, -33.5782)
  line L59 (151.6322, -33.5782) -> (153.2632, -33.5415)
  line L60 (153.2632, -33.5415) -> (155.0015, -39.4872)
  line L61 (155.0015, -39.4872) -> (140.4552, -39.4147)
  line L62 (140.4552, -39.4147) -> (145.2585, -33.5893)
  line L63 (145.2585, -33.5893) -> (145.2588, -33.5908)
  spline S238 degree 3 poles (152.9413, -139.0973) (153.0574, -138.5407) (152.8687, -137.9469) (152.4352, -137.5051) knots 0 0 0 0 1 1 1 1
  spline S239 degree 3 poles (152.4352, -137.5051) (152.0733, -137.1363) (151.5471, -136.8757) (150.9771, -136.783) knots 0 0 0 0 1 1 1 1
  line L64 (150.9771, -136.783) -> (134.7351, -136.4507)
  spline S240 degree 3 poles (134.7351, -136.4507) (134.1896, -136.3913) (133.6161, -136.5275) (133.1964, -136.816) knots 0 0 0 0 1 1 1 1
  spline S241 degree 3 poles (133.1964, -136.816) (132.9356, -136.9952) (132.7339, -137.2302) (132.6173, -137.4907) knots 0 0 0 0 1 1 1 1
  spline S242 degree 3 poles (132.6173, -137.4907) (132.5008, -137.7512) (132.4698, -138.0364) (132.5282, -138.3095) knots 0 0 0 0 1 1 1 1
  line L65 (132.5282, -138.3095) -> (128.64, -202.1235)
  spline S243 degree 3 poles (128.64, -202.1235) (128.6631, -202.7447) (128.9206, -203.359) (129.3692, -203.8632) knots 0 0 0 0 1 1 1 1
  spline S244 degree 3 poles (129.3692, -203.8632) (129.8461, -204.3993) (130.5375, -204.808) (131.3132, -205.0122) knots 0 0 0 0 1 1 1 1
  line L66 (131.3132, -205.0122) -> (185.3432, -208.5574)
  spline S245 degree 3 poles (185.3432, -208.5574) (186.5202, -208.7117) (187.7794, -208.3694) (188.6035, -207.6712) knots 0 0 0 0 1 1 1 1
  spline S246 degree 3 poles (188.6035, -207.6712) (189.0837, -207.2644) (189.4179, -206.7457) (189.5555, -206.1939) knots 0 0 0 0 1 1 1 1
  spline S247 degree 3 poles (189.5555, -206.1939) (191.833, -198.9698) (192.2769, -191.3695) (190.8515, -184.0034) knots 0 0 0 0 1 1 1 1
  spline S248 degree 3 poles (190.8515, -184.0034) (190.588, -182.6414) (190.2528, -181.2667) (189.4827, -180.0374) knots 0 0 0 0 1 1 1 1
  spline S249 degree 3 poles (189.4827, -180.0374) (189.0977, -179.4228) (188.6044, -178.8491) (187.9905, -178.372) knots 0 0 0 0 1 1 1 1
  spline S250 degree 3 poles (187.9905, -178.372) (187.3766, -177.8949) (186.6397, -177.516) (185.8292, -177.3069) knots 0 0 0 0 1 1 1 1
  spline S251 degree 3 poles (185.8292, -177.3069) (184.7984, -177.0409) (183.6823, -177.0562) (182.6184, -177.2149) knots 0 0 0 0 1 1 1 1
  spline S252 degree 3 poles (182.6184, -177.2149) (181.5544, -177.3737) (180.5306, -177.6707) (179.5109, -177.9634) knots 0 0 0 0 1 1 1 1
  spline S253 degree 3 poles (179.5109, -177.9634) (174.1099, -179.5135) (168.6705, -180.9739) (163.229, -182.4277) knots 0 0 0 0 1 1 1 1
  spline S254 degree 3 poles (163.229, -182.4277) (161.8093, -182.807) (160.381, -183.1875) (158.9025, -183.3662) knots 0 0 0 0 1 1 1 1
  spline S255 degree 3 poles (158.9025, -183.3662) (157.424, -183.5448) (155.8785, -183.5131) (154.4804, -183.0843) knots 0 0 0 0 1 1 1 1
  spline S256 degree 3 poles (154.4804, -183.0843) (153.3104, -182.7254) (152.266, -182.0854) (151.5642, -181.2461) knots 0 0 0 0 1 1 1 1
  spline S257 degree 3 poles (151.5642, -181.2461) (150.7386, -180.2587) (150.4116, -179.0058) (150.6732, -177.8321) knots 0 0 0 0 1 1 1 1
  line L67 (150.6732, -177.8321) -> (152.9413, -139.0973)
  line L68 (141.8092, -151.153) -> (144.1576, -148.9711)
  spline S258 degree 3 poles (144.1576, -148.9711) (144.3427, -148.737) (144.4014, -148.4397) (144.3157, -148.1706) knots 0 0 0 0 1 1 1 1
  spline S259 degree 3 poles (144.3157, -148.1706) (144.23, -147.9014) (144.0011, -147.6642) (143.6994, -147.532) knots 0 0 0 0 1 1 1 1
  spline S260 degree 3 poles (143.6994, -147.532) (143.3474, -147.3777) (142.9025, -147.3719) (142.5445, -147.5169) knots 0 0 0 0 1 1 1 1
  spline S261 degree 3 poles (142.5445, -147.5169) (142.1866, -147.662) (141.9253, -147.954) (141.8665, -148.2748) knots 0 0 0 0 1 1 1 1
  spline S262 degree 3 poles (141.8665, -148.2748) (141.849, -148.1147) (141.7807, -147.9584) (141.6702, -147.825) knots 0 0 0 0 1 1 1 1
  spline S263 degree 3 poles (141.6702, -147.825) (141.5596, -147.6915) (141.4069, -147.5812) (141.2307, -147.5075) knots 0 0 0 0 1 1 1 1
  spline S264 degree 3 poles (141.2307, -147.5075) (141.0545, -147.4338) (140.8551, -147.3968) (140.6569, -147.4011) knots 0 0 0 0 1 1 1 1
  spline S265 degree 3 poles (140.6569, -147.4011) (140.4587, -147.405) (140.262, -147.4508) (140.0908, -147.532) knots 0 0 0 0 1 1 1 1
  spline S266 degree 3 poles (140.0908, -147.532) (139.8003, -147.6698) (139.589, -147.9125) (139.5261, -148.1805) knots 0 0 0 0 1 1 1 1
  spline S267 degree 3 poles (139.5261, -148.1805) (139.4633, -148.4485) (139.5501, -148.7372) (139.7581, -148.9517) knots 0 0 0 0 1 1 1 1
  line L69 (139.7581, -148.9517) -> (141.8092, -151.153)
  spline S268 degree 3 poles (172.7469, -194.5735) (172.9307, -194.4863) (173.0796, -194.3515) (173.1661, -194.1938) knots 0 0 0 0 1 1 1 1
  spline S269 degree 3 poles (173.1661, -194.1938) (173.2525, -194.036) (173.2763, -193.8561) (173.2329, -193.6872) knots 0 0 0 0 1 1 1 1
  spline S270 degree 3 poles (173.2329, -193.6872) (173.1892, -193.5169) (173.0776, -193.3586) (172.9188, -193.2417) knots 0 0 0 0 1 1 1 1
  spline S271 degree 3 poles (172.9188, -193.2417) (172.7601, -193.1247) (172.5551, -193.0497) (172.3418, -193.0306) knots 0 0 0 0 1 1 1 1
  line L70 (172.3418, -193.0306) -> (161.5277, -190.7984)
  spline S272 degree 3 poles (161.5277, -190.7984) (161.281, -190.7505) (161.018, -190.7587) (160.7765, -190.822) knots 0 0 0 0 1 1 1 1
  spline S273 degree 3 poles (160.7765, -190.822) (160.5351, -190.8853) (160.316, -191.0035) (160.1506, -191.1595) knots 0 0 0 0 1 1 1 1
  spline S274 degree 3 poles (160.1506, -191.1595) (159.9749, -191.3253) (159.8607, -191.5335) (159.8266, -191.7504) knots 0 0 0 0 1 1 1 1
  line L71 (159.8266, -191.7504) -> (159.7456, -197.0928)
  spline S275 degree 3 poles (159.7456, -197.0928) (159.7601, -197.4387) (160.0025, -197.773) (160.3684, -197.9514) knots 0 0 0 0 1 1 1 1
  spline S276 degree 3 poles (160.3684, -197.9514) (160.5665, -198.0481) (160.7973, -198.1003) (161.0286, -198.1008) knots 0 0 0 0 1 1 1 1
  spline S277 degree 3 poles (161.0286, -198.1008) (161.2598, -198.1013) (161.4909, -198.0501) (161.6898, -197.9544) knots 0 0 0 0 1 1 1 1
  line L72 (161.6898, -197.9544) -> (172.7469, -194.5735)
  spline S278 degree 3 poles (134.2076, -194.4583) (135.0439, -194.804) (136.0062, -194.8821) (136.9441, -194.9155) knots 0 0 0 0 1 1 1 1
  spline S279 degree 3 poles (136.9441, -194.9155) (137.582, -194.9382) (138.221, -194.9431) (138.8593, -194.93) knots 0 0 0 0 1 1 1 1
  line L73 (138.8593, -194.93) -> (139.7185, -193.9551)
  line L74 (139.7185, -193.9551) -> (140.5491, -195.0229)
  spline S280 degree 3 poles (140.5491, -195.0229) (142.4682, -195.0355) (144.3878, -195.0123) (146.3056, -194.9532) knots 0 0 0 0 1 1 1 1
  spline S281 degree 3 poles (146.3056, -194.9532) (147.5238, -194.9157) (148.7462, -194.8633) (149.9428, -194.6747) knots 0 0 0 0 1 1 1 1
  spline S282 degree 3 poles (149.9428, -194.6747) (151.1099, -194.4907) (152.2673, -194.168) (153.2083, -193.5791) knots 0 0 0 0 1 1 1 1
  spline S283 degree 3 poles (153.2083, -193.5791) (153.5103, -193.3901) (153.796, -193.1651) (153.9335, -192.8767) knots 0 0 0 0 1 1 1 1
  spline S284 degree 3 poles (153.9335, -192.8767) (154.0023, -192.7324) (154.0314, -192.5743) (154.0023, -192.4215) knots 0 0 0 0 1 1 1 1
  spline S285 degree 3 poles (154.0023, -192.4215) (153.9732, -192.2687) (153.8837, -192.1219) (153.7415, -192.0189) knots 0 0 0 0 1 1 1 1
  spline S286 degree 3 poles (153.7415, -192.0189) (153.5718, -191.8961) (153.3298, -191.8421) (153.1065, -191.8771) knots 0 0 0 0 1 1 1 1
  line L75 (153.1065, -191.8771) -> (151.0844, -191.981)
  line L76 (151.0844, -191.981) -> (151.0361, -190.6811)
  line L77 (151.0361, -190.6811) -> (150.3763, -190.3748)
  spline S287 degree 3 poles (150.3763, -190.3748) (150.2527, -190.3515) (150.1185, -190.3679) (150.0085, -190.4186) knots 0 0 0 0 1 1 1 1
  spline S288 degree 3 poles (150.0085, -190.4186) (149.8625, -190.4864) (149.7634, -190.6163) (149.7537, -190.7524) knots 0 0 0 0 1 1 1 1
  line L78 (149.7537, -190.7524) -> (149.8286, -192.6088)
  line L79 (149.8286, -192.6088) -> (147.6696, -192.6224)
  line L80 (147.6696, -192.6224) -> (147.5808, -191.4243)
  line L81 (147.5808, -191.4243) -> (147.2802, -191.1733)
  spline S289 degree 3 poles (147.2802, -191.1733) (147.2057, -191.111) (147.1332, -191.0469) (147.0521, -190.9901) knots 0 0 0 0 1 1 1 1
  spline S290 degree 3 poles (147.0521, -190.9901) (146.9711, -190.9334) (146.8765, -190.8848) (146.7705, -190.8726) knots 0 0 0 0 1 1 1 1
  spline S291 degree 3 poles (146.7705, -190.8726) (146.7175, -190.8667) (146.6626, -190.8696) (146.6119, -190.8839) knots 0 0 0 0 1 1 1 1
  spline S292 degree 3 poles (146.6119, -190.8839) (146.5613, -190.898) (146.5153, -190.9229) (146.4797, -190.9552) knots 0 0 0 0 1 1 1 1
  spline S293 degree 3 poles (146.4797, -190.9552) (146.4441, -190.9876) (146.419, -191.0271) (146.4033, -191.0686) knots 0 0 0 0 1 1 1 1
  spline S294 degree 3 poles (146.4033, -191.0686) (146.3877, -191.11) (146.3813, -191.1534) (146.3753, -191.1965) knots 0 0 0 0 1 1 1 1
  line L82 (146.3753, -191.1965) -> (146.338, -191.4708)
  line L83 (146.338, -191.4708) -> (146.2695, -192.7073)
  line L84 (146.2695, -192.7073) -> (143.7284, -192.6892)
  line L85 (143.7284, -192.6892) -> (143.6341, -191.3066)
  spline S295 degree 3 poles (143.6341, -191.3066) (143.649, -191.2198) (143.6193, -191.1287) (143.5533, -191.0593) knots 0 0 0 0 1 1 1 1
  spline S296 degree 3 poles (143.5533, -191.0593) (143.4875, -190.9898) (143.3864, -190.9431) (143.2791, -190.9325) knots 0 0 0 0 1 1 1 1
  spline S297 degree 3 poles (143.2791, -190.9325) (143.1879, -190.9236) (143.0947, -190.9394) (143.0108, -190.9701) knots 0 0 0 0 1 1 1 1
  spline S298 degree 3 poles (143.0108, -190.9701) (142.9268, -191.0004) (142.8513, -191.0441) (142.7803, -191.0915) knots 0 0 0 0 1 1 1 1
  spline S299 degree 3 poles (142.7803, -191.0915) (142.6156, -191.2013) (142.4723, -191.3321) (142.3571, -191.4775) knots 0 0 0 0 1 1 1 1
  line L86 (142.3571, -191.4775) -> (142.2544, -192.5619)
  line L87 (142.2544, -192.5619) -> (141.574, -192.5511)
  spline S300 degree 3 poles (141.574, -192.5511) (141.5328, -192.2008) (141.3567, -191.8618) (141.0765, -191.5932) knots 0 0 0 0 1 1 1 1
  spline S301 degree 3 poles (141.0765, -191.5932) (140.7963, -191.3245) (140.4131, -191.1274) (139.9939, -191.0362) knots 0 0 0 0 1 1 1 1
  spline S302 degree 3 poles (139.9939, -191.0362) (139.4187, -190.9111) (138.7804, -190.9914) (138.2791, -191.2519) knots 0 0 0 0 1 1 1 1
  spline S303 degree 3 poles (138.2791, -191.2519) (137.7778, -191.5123) (137.4213, -191.949) (137.3215, -192.4248) knots 0 0 0 0 1 1 1 1
  line L88 (137.3215, -192.4248) -> (136.6272, -192.4094)
  line L89 (136.6272, -192.4094) -> (136.5483, -191.0128)
  spline S304 degree 3 poles (136.5483, -191.0128) (136.5434, -190.9295) (136.5348, -190.8448) (136.4947, -190.7681) knots 0 0 0 0 1 1 1 1
  spline S305 degree 3 poles (136.4947, -190.7681) (136.4546, -190.6915) (136.3845, -190.6249) (136.296, -190.5825) knots 0 0 0 0 1 1 1 1
  spline S306 degree 3 poles (136.296, -190.5825) (136.2302, -190.551) (136.1521, -190.5336) (136.0765, -190.5428) knots 0 0 0 0 1 1 1 1
  spline S307 degree 3 poles (136.0765, -190.5428) (136.0387, -190.5478) (136.0022, -190.5585) (135.9689, -190.5737) knots 0 0 0 0 1 1 1 1
  spline S308 degree 3 poles (135.9689, -190.5737) (135.9356, -190.5889) (135.9057, -190.6085) (135.876, -190.6281) knots 0 0 0 0 1 1 1 1
  line L90 (135.876, -190.6281) -> (135.3405, -190.9834)
  line L91 (135.3405, -190.9834) -> (135.2601, -192.1761)
  line L92 (135.2601, -192.1761) -> (133.7795, -192.1722)
  spline S309 degree 3 poles (133.7795, -192.1722) (133.471, -192.1909) (133.1775, -192.3327) (133.0103, -192.5437) knots 0 0 0 0 1 1 1 1
  spline S310 degree 3 poles (133.0103, -192.5437) (132.9161, -192.6626) (132.8613, -192.801) (132.8452, -192.9417) knots 0 0 0 0 1 1 1 1
  spline S311 degree 3 poles (132.8452, -192.9417) (132.8291, -193.0824) (132.8512, -193.2253) (132.9029, -193.3602) knots 0 0 0 0 1 1 1 1
  spline S312 degree 3 poles (132.9029, -193.3602) (133.0061, -193.6302) (133.224, -193.8639) (133.4813, -194.0547) knots 0 0 0 0 1 1 1 1
  spline S313 degree 3 poles (133.4813, -194.0547) (133.6985, -194.2158) (133.9454, -194.3498) (134.2076, -194.4583) knots 0 0 0 0 1 1 1 1
  spline S314 degree 3 poles (184.4242, -181.7632) (184.367, -181.7611) (184.3096, -181.7622) (184.2526, -181.7663) knots 0 0 0 0 1 1 1 1
  spline S315 degree 3 poles (184.2526, -181.7663) (183.2204, -182.0053) (183.3818, -182.4234) (183.2753, -183.0369) knots 0 0 0 0 1 1 1 1
  spline S316 degree 3 poles (183.2753, -183.0369) (183.3039, -183.281) (183.2962, -183.6104) (183.3179, -183.9266) knots 0 0 0 0 1 1 1 1
  spline S317 degree 3 poles (183.3179, -183.9266) (182.8674, -183.9544) (182.6952, -183.9088) (182.3172, -183.9489) knots 0 0 0 0 1 1 1 1
  spline S318 degree 3 poles (182.3172, -183.9489) (182.1597, -184.1615) (182.2966, -184.8085) (182.5037, -185.1813) knots 0 0 0 0 1 1 1 1
  spline S319 degree 3 poles (182.5037, -185.1813) (182.8385, -185.3246) (182.9111, -185.2875) (183.2675, -185.2784) knots 0 0 0 0 1 1 1 1
  spline S320 degree 3 poles (183.2675, -185.2784) (183.7573, -185.3089) (183.7861, -185.299) (184.1678, -185.3202) knots 0 0 0 0 1 1 1 1
  spline S321 degree 3 poles (184.1678, -185.3202) (184.2033, -185.937) (184.2096, -185.9768) (184.2568, -187.0119) knots 0 0 0 0 1 1 1 1
  spline S322 degree 3 poles (184.2568, -187.0119) (184.2517, -187.4517) (184.2584, -187.4567) (184.2902, -188.2051) knots 0 0 0 0 1 1 1 1
  spline S323 degree 3 poles (184.2902, -188.2051) (183.7424, -188.2522) (183.5457, -188.245) (183.0656, -188.2741) knots 0 0 0 0 1 1 1 1
  spline S324 degree 3 poles (183.0656, -188.2741) (182.9467, -188.3389) (183.0407, -188.7593) (183.0752, -188.9954) knots 0 0 0 0 1 1 1 1
  spline S325 degree 3 poles (183.0752, -188.9954) (183.2124, -189.4865) (183.1738, -189.4405) (183.7882, -189.4826) knots 0 0 0 0 1 1 1 1